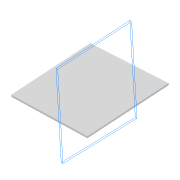
# Autodesk Inventor part: lid2
Saved by Autodesk Inventor 2015 (Build 190159000, 159)
## iProperties
Created: 2015-10-15
Part Number: lid2
Material: Polycarbonate, Clear
Description: insert part description/title
Document SubType Name: Modeling
Designer: c3132704
Density: 1.2 g/cm^3
Appearance: Polycarbonate - Clear
Part Category: insert part category here and press enter to fill value
Author: c3132704
Autodesk Inventor part; units mm, degrees
ref_plane "YZ Plane" through (0, 0, 0) normal (1, 0, 0) x (0, 1, 0)
ref_plane "XZ Plane" through (0, 0, 0) normal (0, 1, 0) x (-1, 0, 0)
ref_plane "XY Plane" through (0, 0, 0) normal (0, 0, 1) x (1, 0, 0)
sketch "Sketch1" plane through (0, 0, 0) normal (0, 0, 1) x (1, 0, 0)
  line L0 (-14.162, 281.2972) -> (-227.9994, 268.0083)
  line L1 (-227.9994, 268.0083) -> (-212.857, 24.346)
  line L2 (-212.857, 24.346) -> (1.4181, 30.5916)
  line L3 (1.4181, 30.5916) -> (-14.162, 281.2972)
  line L4 (-1.2433, 41.1726) -> (-15.9388, 277.6436) construction
  point P0 (0, 0)
  dimension "d6" = 2
  constraints: 8 end point, 1 parallel, 1 perpendicular
  measures "d6" distance between parallel lines of L4 L3
extrude "Extrusion1" add sketch "Sketch1" along normal blind 5
body "Solid1"
